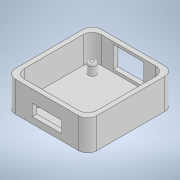
# Autodesk Inventor part: micro lipo case
Saved by Autodesk Inventor 2020 (Build 240168000, 168)
## iProperties
Created: 2020-08-31
Part Number: micro lipo case
Material: Generic
Document SubType Name: Modeling
Designer: mulve
Density: 1 g/cm^3
Appearance: Default
Author: mulve
Autodesk Inventor part; units mm, degrees
ref_plane "YZ Plane" through (0, 0, 0) normal (1, 0, 0) x (0, 1, 0)
ref_plane "XZ Plane" through (0, 0, 0) normal (0, 1, 0) x (-1, 0, 0)
ref_plane "XY Plane" through (0, 0, 0) normal (0, 0, 1) x (1, 0, 0)
sketch "Sketch1" plane through (0, 0, 0) normal (0, 1, 0) x (-1, 0, 0)
  line L0 (0, 0) -> (22.86, 0)
  line L1 (22.86, 0) -> (22.86, -24.13)
  line L2 (22.86, -24.13) -> (0, -24.13)
  line L3 (0, -24.13) -> (0, 0)
  dimension "d0" = 24.13
  dimension "d1" = 22.86
  constraints: 8 end point, 2 parallel, 1 horizontal, 1 perpendicular
  measures "d0" distance of L0.end L1.end
  measures "d1" distance of L1.end L2.end
extrude "Extrusion1" add sketch "Sketch1" along normal blind 8.5
sketch "Sketch2" plane through (0, 8.5, 0) normal (0, 1, 0) x (1, 0, 0)
  line L0 (-1.27, 1.27) -> (-21.59, 1.27)
  line L1 (-21.59, 1.27) -> (-21.59, 22.86)
  line L2 (-21.59, 22.86) -> (-1.27, 22.86)
  line L3 (-1.27, 22.86) -> (-1.27, 1.27)
  line L4 (-22.86, 0) -> (0, 0) projected
  line L5 (0, 24.13) -> (-22.86, 24.13) projected
  line L6 (0, 0) -> (0, 24.13) projected
  line L7 (-22.86, 24.13) -> (-22.86, 0) projected
  dimension "d4" = 21.59
  dimension "d5" = 20.32
  dimension "d6" = 1.27
  dimension "d7" = 1.27
  dimension "d8" = 1.27
  dimension "d9" = 1.27
  constraints: 8 end point, 2 parallel, 1 horizontal, 1 perpendicular
  measures "d4" distance of L0.end L1.end
  measures "d5" distance of L1.end L2.end
  measures "d6" distance between parallel lines of L4 L0
  measures "d7" distance between parallel lines of L5 L2
  measures "d8" distance between parallel lines of L6 L3
  measures "d9" distance between parallel lines of L7 L1
extrude "Extrusion2" cut sketch "Sketch2" against normal blind 7.5 contours L0 L1 L2 L3
fillet "Fillet1" radius 2.54 4 edges at (-21.59, 4.75, -1.27) (-21.59, 4.75, -22.86) (-1.27, 4.75, -22.86) (-1.27, 4.75, -1.27)
sketch "Sketch3" plane through (0, 1, 0) normal (0, 1, 0) x (1, 0, 0)
  line L0 (-3.81, 1.27) -> (-19.05, 1.27) projected
  line L1 (-19.05, 22.86) -> (-3.81, 22.86) projected
  line L2 (-1.27, 20.32) -> (-1.27, 3.81) projected
  line L3 (-21.59, 3.81) -> (-21.59, 20.32) projected
  circle A0 centre (-18.415, 4.445) radius 1.0795
  circle A1 centre (-18.415, 19.685) radius 1.0795
  circle A2 centre (-4.445, 19.685) radius 1.0795
  circle A3 centre (-4.445, 4.445) radius 1.0795
  point P0 (0, 0)
  dimension "d13" = 13.97
  dimension "d14" = 15.24
  dimension "d15" = 13.97
  dimension "d16" = 15.24
  dimension "d17" = 3.175
  dimension "d19" = 3.175
  dimension "d20" = 3.175
  dimension "d21" = 3.175
  dimension "d22" = 3.175
  dimension "d23" = 3.175
  dimension "d24" = 2.159
  constraints: 4 centre point, 3 coincident, 3 equal radius
  measures "d13" distance of point (-4.445, 4.445) point (-18.415, 4.445)
  measures "d14" distance of point (-4.445, 19.685) point (-4.445, 4.445)
  measures "d15" distance of point (-18.415, 19.685) point (-4.445, 19.685)
  measures "d16" distance of point (-18.415, 4.445) point (-18.415, 19.685)
  measures "d17" distance from line of L0 point (-4.445, 4.445)
  measures "d19" distance from line of L1 point (-4.445, 19.685)
  measures "d20" distance from line of L0 point (-18.415, 4.445)
  measures "d21" distance from line of L1 point (-18.415, 19.685)
  measures "d22" distance from line of L2 point (-4.445, 19.685)
  measures "d23" distance from line of L3 point (-18.415, 19.685)
  measures "d24" diameter of A0
extrude "Extrusion3" add sketch "Sketch3" along normal blind 3
fillet "Fillet2" radius 0.635 4 edges at (-19.4945, 4, -19.685) (-5.5245, 4, -19.685) (-19.4945, 4, -4.445) (-5.5245, 4, -4.445)
sketch "Sketch4" plane through (-22.86, 0, 0) normal (0, 0, 1) x (1, 0, 0)
  line L0 (7.305, 5.025) -> (15.555, 5.025)
  line L1 (15.555, 5.025) -> (15.555, 1.775)
  line L2 (15.555, 1.775) -> (7.305, 1.775)
  line L3 (7.305, 1.775) -> (7.305, 5.025)
  line L4 (0, 0) -> (0, 8.5) projected
  line L5 (22.86, 0) -> (22.86, 8.5) projected
  line L6 (19.05, 1) -> (3.81, 1) projected
  dimension "d28" = 8.25
  dimension "d29" = 3.25
  dimension "d30" = 7.305
  dimension "d31" = 7.305
  dimension "d32" = 0.775
  constraints: 8 end point, 2 parallel, 1 horizontal, 1 perpendicular
  measures "d28" distance of L0.start L0.end
  measures "d29" distance of L2.end L0.start
  measures "d30" distance between parallel lines of L4 L3
  measures "d31" distance between parallel lines of L5 L1
  measures "d32" distance between parallel lines of L6 L2
extrude "Extrusion4" cut sketch "Sketch4" against normal up to surface (1.27 mm away)
sketch "Sketch5" plane through (0, 0, -24.13) normal (0, 0, -1) x (-1, 0, 0)
  line L0 (7.18, 7.775) -> (15.68, 7.775)
  line L1 (15.68, 7.775) -> (15.68, 1.775)
  line L2 (15.68, 1.775) -> (7.18, 1.775)
  line L3 (7.18, 1.775) -> (7.18, 7.775)
  line L4 (0, 0) -> (0, 8.5) projected
  line L5 (22.86, 0) -> (22.86, 8.5) projected
  line L6 (0, 0) -> (22.86, 0) projected
  line L7 (19.05, 1) -> (3.81, 1) projected
  dimension "d35" = 8.5
  dimension "d36" = 6
  dimension "d37" = 7.18
  dimension "d38" = 7.18
  dimension "d43" = 0.775
  constraints: 8 end point, 2 parallel, 1 horizontal, 1 perpendicular
  measures "d35" distance of L0.start L0.end
  measures "d36" distance of L2.end L0.start
  measures "d37" distance between parallel lines of L4 L3
  measures "d38" distance between parallel lines of L5 L1
  measures "d43" distance between parallel lines of L7 L2
extrude "Extrusion5" cut sketch "Sketch5" against normal up to surface (1.27 mm away)
fillet "Fillet3" radius 2.54 4 edges at (0, 4.25, 0) (-22.86, 4.25, 0) (0, 4.25, -24.13) (-22.86, 4.25, -24.13)
equation "\"d6\" = d7"
equation "\"d8\" = d9"
equation "\"d16\" = d14"
equation "\"d22\" = d23"
equation "\"d30\" = d31"
equation "\"d37\" = d38"
body "Solid1"
